Autodesk Fusion 360 part; units mm, degrees
(part 7 of 9)
  spline S163 degree 3 poles (2.1351, 29.8276) (2.5485, 29.4473) (2.7552, 28.9129) (2.7552, 28.2236) knots 0 0 0 0 1 1 1 1
  spline S164 degree 3 poles (2.7552, 28.2236) (2.7552, 27.6314) (2.5712, 27.1156) (2.2023, 26.6753) knots 0 0 0 0 1 1 1 1
  spline S165 degree 3 poles (2.2023, 26.6753) (1.8333, 26.2361) (1.2669, 26.017) (0.5021, 26.017) knots 0 0 0 0 1 1 1 1
  line L345 (0.5021, 26.017) -> (-1.8853, 26.017)
  line L346 (-1.8853, 26.017) -> (-1.8853, 22.8079)
  line L347 (-1.8853, 22.8079) -> (-2.9137, 22.8079)
  line L348 (-2.9137, 22.8079) -> (-2.9137, 30.3992)
  spline S166 degree 3 poles (1.7165, 28.2184) (1.7165, 28.7765) (1.5098, 29.1558) (1.0964, 29.3553) knots 0 0 0 0 1 1 1 1
  spline S167 degree 3 poles (1.0964, 29.3553) (0.869, 29.4617) (0.5569, 29.5155) (0.161, 29.5155) knots 0 0 0 0 1 1 1 1
  line L349 (0.161, 29.5155) -> (-1.8853, 29.5155)
  line L350 (-1.8853, 29.5155) -> (-1.8853, 26.8852)
  line L351 (-1.8853, 26.8852) -> (0.161, 26.8852)
  spline S168 degree 3 poles (0.161, 26.8852) (0.623, 26.8852) (0.9972, 26.9833) (1.2855, 27.1797) knots 0 0 0 0 1 1 1 1
  spline S169 degree 3 poles (1.2855, 27.1797) (1.5728, 27.3761) (1.7165, 27.7223) (1.7165, 28.2184) knots 0 0 0 0 1 1 1 1
  line L352 (13.755, 30.3992) -> (17.1709, 30.3992)
  spline S170 degree 3 poles (17.1709, 30.3992) (17.8458, 30.3992) (18.3904, 30.209) (18.8038, 29.8276) knots 0 0 0 0 1 1 1 1
  spline S171 degree 3 poles (18.8038, 29.8276) (19.2172, 29.4473) (19.424, 28.9129) (19.424, 28.2236) knots 0 0 0 0 1 1 1 1
  spline S172 degree 3 poles (19.424, 28.2236) (19.424, 27.6314) (19.24, 27.1156) (18.871, 26.6753) knots 0 0 0 0 1 1 1 1
  spline S173 degree 3 poles (18.871, 26.6753) (18.502, 26.2361) (17.9357, 26.017) (17.1709, 26.017) knots 0 0 0 0 1 1 1 1
  line L353 (17.1709, 26.017) -> (14.7834, 26.017)
  line L354 (14.7834, 26.017) -> (14.7834, 22.8079)
  line L355 (14.7834, 22.8079) -> (13.755, 22.8079)
  line L356 (13.755, 22.8079) -> (13.755, 30.3992)
  spline S174 degree 3 poles (18.3853, 28.2184) (18.3853, 28.7765) (18.1785, 29.1558) (17.7651, 29.3553) knots 0 0 0 0 1 1 1 1
  spline S175 degree 3 poles (17.7651, 29.3553) (17.5378, 29.4617) (17.2256, 29.5155) (16.8298, 29.5155) knots 0 0 0 0 1 1 1 1
  line L357 (16.8298, 29.5155) -> (14.7834, 29.5155)
  line L358 (14.7834, 29.5155) -> (14.7834, 26.8852)
  line L359 (14.7834, 26.8852) -> (16.8298, 26.8852)
  spline S176 degree 3 poles (16.8298, 26.8852) (17.2918, 26.8852) (17.6659, 26.9833) (17.9543, 27.1797) knots 0 0 0 0 1 1 1 1
  spline S177 degree 3 poles (17.9543, 27.1797) (18.2416, 27.3761) (18.3853, 27.7223) (18.3853, 28.2184) knots 0 0 0 0 1 1 1 1
  line L360 (29.7365, 30.3992) -> (30.9354, 30.3992)
  line L361 (30.9354, 30.3992) -> (33.1161, 26.7508)
  line L362 (33.1161, 26.7508) -> (35.2969, 30.3992)
  line L363 (35.2969, 30.3992) -> (36.5009, 30.3992)
  line L364 (36.5009, 30.3992) -> (33.6329, 25.8671)
  line L365 (33.6329, 25.8671) -> (33.6329, 22.8079)
  line L366 (33.6329, 22.8079) -> (32.6045, 22.8079)
  line L367 (32.6045, 22.8079) -> (32.6045, 25.8671)
  line L368 (32.6045, 25.8671) -> (29.7365, 30.3992)
  line L369 (47.5938, 30.3992) -> (49.7746, 23.9344)
  line L370 (49.7746, 23.9344) -> (51.9295, 30.3992)
  line L371 (51.9295, 30.3992) -> (53.0818, 30.3992)
  line L372 (53.0818, 30.3992) -> (50.312, 22.8079)
  line L373 (50.312, 22.8079) -> (49.2216, 22.8079)
  line L374 (49.2216, 22.8079) -> (46.4569, 30.3992)
  line L375 (46.4569, 30.3992) -> (47.5938, 30.3992)
  spline S178 degree 3 poles (66.3534, 30.6059) (67.6939, 30.6059) (68.6861, 30.1749) (69.3299, 29.3139) knots 0 0 0 0 1 1 1 1
  spline S179 degree 3 poles (69.3299, 29.3139) (69.8333, 28.6422) (70.0844, 27.7823) (70.0844, 26.7353) knots 0 0 0 0 1 1 1 1
  spline S180 degree 3 poles (70.0844, 26.7353) (70.0844, 25.6015) (69.7971, 24.66) (69.2214, 23.9086) knots 0 0 0 0 1 1 1 1
  spline S181 degree 3 poles (69.2214, 23.9086) (68.5465, 23.027) (67.5833, 22.5857) (66.3327, 22.5857) knots 0 0 0 0 1 1 1 1
  spline S182 degree 3 poles (66.3327, 22.5857) (65.1648, 22.5857) (64.2471, 22.9712) (63.5784, 23.7432) knots 0 0 0 0 1 1 1 1
  spline S183 degree 3 poles (63.5784, 23.7432) (62.982, 24.4874) (62.6844, 25.4279) (62.6844, 26.5648) knots 0 0 0 0 1 1 1 1
  spline S184 degree 3 poles (62.6844, 26.5648) (62.6844, 27.5911) (62.9396, 28.4696) (63.4492, 29.2003) knots 0 0 0 0 1 1 1 1
  spline S185 degree 3 poles (63.4492, 29.2003) (64.1034, 30.1377) (65.0718, 30.6059) (66.3534, 30.6059) knots 0 0 0 0 1 1 1 1
  spline S186 degree 3 poles (66.4567, 23.5055) (67.3631, 23.5055) (68.0184, 23.83) (68.4225, 24.4801) knots 0 0 0 0 1 1 1 1
  spline S187 degree 3 poles (68.4225, 24.4801) (68.8277, 25.1292) (69.0302, 25.8754) (69.0302, 26.7198) knots 0 0 0 0 1 1 1 1
  spline S188 degree 3 poles (69.0302, 26.7198) (69.0302, 27.6117) (68.7966, 28.33) (68.3295, 28.8747) knots 0 0 0 0 1 1 1 1
  spline S189 degree 3 poles (68.3295, 28.8747) (67.8634, 29.4194) (67.2247, 29.6912) (66.4154, 29.6912) knots 0 0 0 0 1 1 1 1
  spline S190 degree 3 poles (66.4154, 29.6912) (65.6299, 29.6912) (64.9891, 29.4214) (64.493, 28.883) knots 0 0 0 0 1 1 1 1
  spline S191 degree 3 poles (64.493, 28.883) (63.9969, 28.3435) (63.7489, 27.5487) (63.7489, 26.4976) knots 0 0 0 0 1 1 1 1
  spline S192 degree 3 poles (63.7489, 26.4976) (63.7489, 25.6573) (63.9618, 24.9483) (64.3876, 24.3706) knots 0 0 0 0 1 1 1 1
  spline S193 degree 3 poles (64.3876, 24.3706) (64.8124, 23.7939) (65.5028, 23.5055) (66.4567, 23.5055) knots 0 0 0 0 1 1 1 1
  spline S194 degree 3 poles (83.5689, 26.9213) (84.0515, 26.9213) (84.4329, 27.0174) (84.713, 27.2107) knots 0 0 0 0 1 1 1 1
  spline S195 degree 3 poles (84.713, 27.2107) (84.9941, 27.404) (85.1347, 27.7513) (85.1347, 28.2546) knots 0 0 0 0 1 1 1 1
  spline S196 degree 3 poles (85.1347, 28.2546) (85.1347, 28.7951) (84.9383, 29.1641) (84.5456, 29.3605) knots 0 0 0 0 1 1 1 1
  spline S197 degree 3 poles (84.5456, 29.3605) (84.3358, 29.4638) (84.0546, 29.5155) (83.7032, 29.5155) knots 0 0 0 0 1 1 1 1
  line L376 (83.7032, 29.5155) -> (81.1918, 29.5155)
  line L377 (81.1918, 29.5155) -> (81.1918, 26.9213)
  line L378 (81.1918, 26.9213) -> (83.5689, 26.9213)
  line L379 (80.1634, 30.3992) -> (83.6774, 30.3992)
  spline S198 degree 3 poles (83.6774, 30.3992) (84.2562, 30.3992) (84.7337, 30.3144) (85.1088, 30.1459) knots 0 0 0 0 1 1 1 1
  spline S199 degree 3 poles (85.1088, 30.1459) (85.822, 29.8224) (86.1785, 29.224) (86.1785, 28.3528) knots 0 0 0 0 1 1 1 1
  spline S200 degree 3 poles (86.1785, 28.3528) (86.1785, 27.898) (86.0845, 27.5259) (85.8974, 27.2366) knots 0 0 0 0 1 1 1 1
  spline S201 degree 3 poles (85.8974, 27.2366) (85.7093, 26.9472) (85.4468, 26.7146) (85.1088, 26.5389) knots 0 0 0 0 1 1 1 1
  spline S202 degree 3 poles (85.1088, 26.5389) (85.4055, 26.418) (85.6287, 26.2599) (85.7775, 26.0635) knots 0 0 0 0 1 1 1 1
  spline S203 degree 3 poles (85.7775, 26.0635) (85.9274, 25.8671) (86.0111, 25.5488) (86.0287, 25.1075) knots 0 0 0 0 1 1 1 1
  line L380 (86.0287, 25.1075) -> (86.0648, 24.0895)
  spline S204 degree 3 poles (86.0648, 24.0895) (86.0752, 23.8001) (86.099, 23.5851) (86.1372, 23.4435) knots 0 0 0 0 1 1 1 1
  spline S205 degree 3 poles (86.1372, 23.4435) (86.1992, 23.2027) (86.3098, 23.0477) (86.4679, 22.9784) knots 0 0 0 0 1 1 1 1
  line L381 (86.4679, 22.9784) -> (86.4679, 22.8079)
  line L382 (86.4679, 22.8079) -> (85.207, 22.8079)
  spline S206 degree 3 poles (85.207, 22.8079) (85.1729, 22.873) (85.145, 22.9577) (85.1243, 23.0611) knots 0 0 0 0 1 1 1 1
  spline S207 degree 3 poles (85.1243, 23.0611) (85.1037, 23.1645) (85.0861, 23.3639) (85.0727, 23.6605) knots 0 0 0 0 1 1 1 1
  line L383 (85.0727, 23.6605) -> (85.0106, 24.9266)
  spline S208 degree 3 poles (85.0106, 24.9266) (84.9869, 25.4227) (84.8019, 25.7555) (84.4577, 25.924) knots 0 0 0 0 1 1 1 1
  spline S209 degree 3 poles (84.4577, 25.924) (84.2613, 26.017) (83.9533, 26.0635) (83.5327, 26.0635) knots 0 0 0 0 1 1 1 1
  line L384 (83.5327, 26.0635) -> (81.1918, 26.0635)
  line L385 (81.1918, 26.0635) -> (81.1918, 22.8079)
  line L386 (81.1918, 22.8079) -> (80.1634, 22.8079)
  line L387 (80.1634, 22.8079) -> (80.1634, 30.3992)
  line L388 (-86.6223, 11.899) -> (-85.5836, 11.899)
  line L389 (-85.5836, 11.899) -> (-85.5836, 8.7622)
  line L390 (-85.5836, 8.7622) -> (-81.6355, 8.7622)
  line L391 (-81.6355, 8.7622) -> (-81.6355, 11.899)
  line L392 (-81.6355, 11.899) -> (-80.5968, 11.899)
  line L393 (-80.5968, 11.899) -> (-80.5968, 4.3077)
  line L394 (-80.5968, 4.3077) -> (-81.6355, 4.3077)
  line L395 (-81.6355, 4.3077) -> (-81.6355, 7.8579)
  line L396 (-81.6355, 7.8579) -> (-85.5836, 7.8579)
  line L397 (-85.5836, 7.8579) -> (-85.5836, 4.3077)
  line L398 (-85.5836, 4.3077) -> (-86.6223, 4.3077)
  line L399 (-86.6223, 4.3077) -> (-86.6223, 11.899)
  line L400 (-65.7905, 7.4186) -> (-66.9429, 10.7724)
  line L401 (-66.9429, 10.7724) -> (-68.1676, 7.4186)
  line L402 (-68.1676, 7.4186) -> (-65.7905, 7.4186)
  line L403 (-67.4803, 11.899) -> (-66.3176, 11.899)
  line L404 (-66.3176, 11.899) -> (-63.5632, 4.3077)
  line L405 (-63.5632, 4.3077) -> (-64.6898, 4.3077)
  line L406 (-64.6898, 4.3077) -> (-65.4598, 6.5815)
  line L407 (-65.4598, 6.5815) -> (-68.4622, 6.5815)
  line L408 (-68.4622, 6.5815) -> (-69.2838, 4.3077)
  line L409 (-69.2838, 4.3077) -> (-70.338, 4.3077)
  line L410 (-70.338, 4.3077) -> (-67.4803, 11.899)
  line L411 (-52.4321, 11.899) -> (-51.4038, 11.899)
  line L412 (-51.4038, 11.899) -> (-51.4038, 5.2121)
  line L413 (-51.4038, 5.2121) -> (-47.559, 5.2121)
  line L414 (-47.559, 5.2121) -> (-47.559, 4.3077)
  line L415 (-47.559, 4.3077) -> (-52.4321, 4.3077)
  line L416 (-52.4321, 4.3077) -> (-52.4321, 11.899)
  spline S210 degree 3 poles (-33.4969, 8.6899) (-33.0628, 8.6899) (-32.7248, 8.7498) (-32.484, 8.8708) knots 0 0 0 0 1 1 1 1
  spline S211 degree 3 poles (-32.484, 8.8708) (-32.1047, 9.0599) (-31.9156, 9.401) (-31.9156, 9.8939) knots 0 0 0 0 1 1 1 1
  spline S212 degree 3 poles (-31.9156, 9.8939) (-31.9156, 10.39) (-32.1171, 10.7239) (-32.5202, 10.8965) knots 0 0 0 0 1 1 1 1
  spline S213 degree 3 poles (-32.5202, 10.8965) (-32.7475, 10.9926) (-33.0855, 11.0412) (-33.533, 11.0412) knots 0 0 0 0 1 1 1 1
  line L417 (-33.533, 11.0412) -> (-35.3675, 11.0412)
  line L418 (-35.3675, 11.0412) -> (-35.3675, 8.6899)
  line L419 (-35.3675, 8.6899) -> (-33.4969, 8.6899)
  spline S214 degree 3 poles (-33.1506, 5.1862) (-32.5202, 5.1862) (-32.0706, 5.3692) (-31.8019, 5.734) knots 0 0 0 0 1 1 1 1
  spline S215 degree 3 poles (-31.8019, 5.734) (-31.6334, 5.9645) (-31.5486, 6.2435) (-31.5486, 6.5712) knots 0 0 0 0 1 1 1 1
  spline S216 degree 3 poles (-31.5486, 6.5712) (-31.5486, 7.122) (-31.7946, 7.4982) (-32.2876, 7.6977) knots 0 0 0 0 1 1 1 1
  spline S217 degree 3 poles (-32.2876, 7.6977) (-32.5491, 7.8042) (-32.8953, 7.8579) (-33.3263, 7.8579) knots 0 0 0 0 1 1 1 1
  line L420 (-33.3263, 7.8579) -> (-35.3675, 7.8579)
  line L421 (-35.3675, 7.8579) -> (-35.3675, 5.1862)
  line L422 (-35.3675, 5.1862) -> (-33.1506, 5.1862)
  line L423 (-36.3752, 11.899) -> (-33.1144, 11.899)
  spline S218 degree 3 poles (-33.1144, 11.899) (-32.2256, 11.899) (-31.5931, 11.6334) (-31.2179, 11.1032) knots 0 0 0 0 1 1 1 1
  spline S219 degree 3 poles (-31.2179, 11.1032) (-30.9978, 10.79) (-30.8872, 10.4283) (-30.8872, 10.018) knots 0 0 0 0 1 1 1 1
  spline S220 degree 3 poles (-30.8872, 10.018) (-30.8872, 9.5394) (-31.0236, 9.1467) (-31.2954, 8.8397) knots 0 0 0 0 1 1 1 1
  spline S221 degree 3 poles (-31.2954, 8.8397) (-31.437, 8.6775) (-31.6396, 8.5297) (-31.9052, 8.3953) knots 0 0 0 0 1 1 1 1
  spline S222 degree 3 poles (-31.9052, 8.3953) (-31.5156, 8.2475) (-31.2252, 8.0801) (-31.0319, 7.8941) knots 0 0 0 0 1 1 1 1
  spline S223 degree 3 poles (-31.0319, 7.8941) (-30.6908, 7.5633) (-30.5203, 7.1065) (-30.5203, 6.5246) knots 0 0 0 0 1 1 1 1
  spline S224 degree 3 poles (-30.5203, 6.5246) (-30.5203, 6.0358) (-30.6733, 5.5924) (-30.9802, 5.1966) knots 0 0 0 0 1 1 1 1
  spline S225 degree 3 poles (-30.9802, 5.1966) (-31.4381, 4.6043) (-32.1667, 4.3077) (-33.1661, 4.3077) knots 0 0 0 0 1 1 1 1
  line L424 (-33.1661, 4.3077) -> (-36.3752, 4.3077)
  line L425 (-36.3752, 4.3077) -> (-36.3752, 11.899)
  line L426 (-17.3883, 11.899) -> (-16.3496, 11.899)
  line L427 (-16.3496, 11.899) -> (-16.3496, 4.3077)
  line L428 (-16.3496, 4.3077) -> (-17.3883, 4.3077)
  line L429 (-17.3883, 4.3077) -> (-17.3883, 11.899)
  spline S226 degree 3 poles (0.2251, 8.4212) (0.7078, 8.4212) (1.0892, 8.5173) (1.3692, 8.7106) knots 0 0 0 0 1 1 1 1
  spline S227 degree 3 poles (1.3692, 8.7106) (1.6504, 8.9038) (1.7909, 9.2511) (1.7909, 9.7544) knots 0 0 0 0 1 1 1 1
  spline S228 degree 3 poles (1.7909, 9.7544) (1.7909, 10.295) (1.5945, 10.6639) (1.2018, 10.8603) knots 0 0 0 0 1 1 1 1
  spline S229 degree 3 poles (1.2018, 10.8603) (0.992, 10.9636) (0.7109, 11.0153) (0.3595, 11.0153) knots 0 0 0 0 1 1 1 1
  line L430 (0.3595, 11.0153) -> (-2.152, 11.0153)
  line L431 (-2.152, 11.0153) -> (-2.152, 8.4212)
  line L432 (-2.152, 8.4212) -> (0.2251, 8.4212)
  line L433 (-3.1804, 11.899) -> (0.3336, 11.899)
  spline S230 degree 3 poles (0.3336, 11.899) (0.9124, 11.899) (1.3899, 11.8142) (1.7651, 11.6458) knots 0 0 0 0 1 1 1 1
  spline S231 degree 3 poles (1.7651, 11.6458) (2.4782, 11.3223) (2.8348, 10.7239) (2.8348, 9.8526) knots 0 0 0 0 1 1 1 1
  spline S232 degree 3 poles (2.8348, 9.8526) (2.8348, 9.3979) (2.7407, 9.0258) (2.5537, 8.7364) knots 0 0 0 0 1 1 1 1
  spline S233 degree 3 poles (2.5537, 8.7364) (2.3656, 8.447) (2.103, 8.2145) (1.7651, 8.0388) knots 0 0 0 0 1 1 1 1
  spline S234 degree 3 poles (1.7651, 8.0388) (2.0617, 7.9178) (2.2849, 7.7597) (2.4338, 7.5633) knots 0 0 0 0 1 1 1 1
  spline S235 degree 3 poles (2.4338, 7.5633) (2.5836, 7.367) (2.6674, 7.0486) (2.6849, 6.6073) knots 0 0 0 0 1 1 1 1
  line L434 (2.6849, 6.6073) -> (2.7211, 5.5893)
  spline S236 degree 3 poles (2.7211, 5.5893) (2.7314, 5.2999) (2.7552, 5.0849) (2.7934, 4.9433) knots 0 0 0 0 1 1 1 1
  spline S237 degree 3 poles (2.7934, 4.9433) (2.8555, 4.7025) (2.966, 4.5475) (3.1242, 4.4783) knots 0 0 0 0 1 1 1 1
  line L435 (3.1242, 4.4783) -> (3.1242, 4.3077)
  line L436 (3.1242, 4.3077) -> (1.8633, 4.3077)
  spline S238 degree 3 poles (1.8633, 4.3077) (1.8292, 4.3728) (1.8013, 4.4576) (1.7806, 4.5609) knots 0 0 0 0 1 1 1 1
  spline S239 degree 3 poles (1.7806, 4.5609) (1.7599, 4.6643) (1.7423, 4.8638) (1.7289, 5.1604) knots 0 0 0 0 1 1 1 1
  line L437 (1.7289, 5.1604) -> (1.6669, 6.4265)
  spline S240 degree 3 poles (1.6669, 6.4265) (1.6431, 6.9226) (1.4581, 7.2553) (1.114, 7.4238) knots 0 0 0 0 1 1 1 1
  spline S241 degree 3 poles (1.114, 7.4238) (0.9176, 7.5168) (0.6096, 7.5633) (0.1889, 7.5633) knots 0 0 0 0 1 1 1 1
  line L438 (0.1889, 7.5633) -> (-2.152, 7.5633)
  line L439 (-2.152, 7.5633) -> (-2.152, 4.3077)
  line L440 (-2.152, 4.3077) -> (-3.1804, 4.3077)
  line L441 (-3.1804, 4.3077) -> (-3.1804, 11.899)
  line L442 (19.4777, 11.899) -> (19.4777, 10.9947)
  line L443 (19.4777, 10.9947) -> (16.9197, 10.9947)
  line L444 (16.9197, 10.9947) -> (16.9197, 4.3077)
  line L445 (16.9197, 4.3077) -> (15.8758, 4.3077)
  line L446 (15.8758, 4.3077) -> (15.8758, 10.9947)
  line L447 (15.8758, 10.9947) -> (13.3179, 10.9947)
  line L448 (13.3179, 10.9947) -> (13.3179, 11.899)
  line L449 (13.3179, 11.899) -> (19.4777, 11.899)
  line L450 (30.059, 11.899) -> (31.0977, 11.899)
  line L451 (31.0977, 11.899) -> (31.0977, 8.7622)
  line L452 (31.0977, 8.7622) -> (35.0457, 8.7622)
  line L453 (35.0457, 8.7622) -> (35.0457, 11.899)
  line L454 (35.0457, 11.899) -> (36.0844, 11.899)
  line L455 (36.0844, 11.899) -> (36.0844, 4.3077)
  line L456 (36.0844, 4.3077) -> (35.0457, 4.3077)
  line L457 (35.0457, 4.3077) -> (35.0457, 7.8579)
  line L458 (35.0457, 7.8579) -> (31.0977, 7.8579)
  line L459 (31.0977, 7.8579) -> (31.0977, 4.3077)
  line L460 (31.0977, 4.3077) -> (30.059, 4.3077)
  line L461 (30.059, 4.3077) -> (30.059, 11.899)
  spline S242 degree 3 poles (49.6164, 5.1862) (49.9647, 5.1862) (50.25, 5.2224) (50.4743, 5.2947) knots 0 0 0 0 1 1 1 1
  spline S243 degree 3 poles (50.4743, 5.2947) (50.8742, 5.4291) (51.2008, 5.6875) (51.4561, 6.0699) knots 0 0 0 0 1 1 1 1
  spline S244 degree 3 poles (51.4561, 6.0699) (51.6597, 6.3768) (51.8054, 6.7696) (51.8954, 7.2481) knots 0 0 0 0 1 1 1 1
  spline S245 degree 3 poles (51.8954, 7.2481) (51.947, 7.5344) (51.9729, 7.799) (51.9729, 8.0439) knots 0 0 0 0 1 1 1 1
  spline S246 degree 3 poles (51.9729, 8.0439) (51.9729, 8.9844) (51.7858, 9.7151) (51.4127, 10.235) knots 0 0 0 0 1 1 1 1
  spline S247 degree 3 poles (51.4127, 10.235) (51.0386, 10.7549) (50.436, 11.0153) (49.6061, 11.0153) knots 0 0 0 0 1 1 1 1
  line L462 (49.6061, 11.0153) -> (47.7819, 11.0153)
  line L463 (47.7819, 11.0153) -> (47.7819, 5.1862)
  line L464 (47.7819, 5.1862) -> (49.6164, 5.1862)
  line L465 (46.7484, 11.899) -> (49.8231, 11.899)
  spline S248 degree 3 poles (49.8231, 11.899) (50.867, 11.899) (51.6762, 11.529) (52.2519, 10.7879) knots 0 0 0 0 1 1 1 1
  spline S249 degree 3 poles (52.2519, 10.7879) (52.7656, 10.1193) (53.0219, 9.2635) (53.0219, 8.2196) knots 0 0 0 0 1 1 1 1
  spline S250 degree 3 poles (53.0219, 8.2196) (53.0219, 7.4135) (52.87, 6.6848) (52.5671, 6.0337) knots 0 0 0 0 1 1 1 1
  spline S251 degree 3 poles (52.5671, 6.0337) (52.0328, 4.8834) (51.115, 4.3077) (49.8128, 4.3077) knots 0 0 0 0 1 1 1 1
  line L466 (49.8128, 4.3077) -> (46.7484, 4.3077)
  line L467 (46.7484, 4.3077) -> (46.7484, 11.899)
  line L468 (67.5595, 7.4186) -> (66.4071, 10.7724)
  line L469 (66.4071, 10.7724) -> (65.1824, 7.4186)
  line L470 (65.1824, 7.4186) -> (67.5595, 7.4186)
  line L471 (65.8697, 11.899) -> (67.0324, 11.899)
  line L472 (67.0324, 11.899) -> (69.7868, 4.3077)
  line L473 (69.7868, 4.3077) -> (68.6602, 4.3077)
  line L474 (68.6602, 4.3077) -> (67.8902, 6.5815)
  line L475 (67.8902, 6.5815) -> (64.8878, 6.5815)
  line L476 (64.8878, 6.5815) -> (64.0662, 4.3077)
  line L477 (64.0662, 4.3077) -> (63.012, 4.3077)
  line L478 (63.012, 4.3077) -> (65.8697, 11.899)
  line L479 (79.7427, 11.899) -> (80.9416, 11.899)
  line L480 (80.9416, 11.899) -> (83.1224, 8.2506)
  line L481 (83.1224, 8.2506) -> (85.3031, 11.899)
  line L482 (85.3031, 11.899) -> (86.5072, 11.899)
  line L483 (86.5072, 11.899) -> (83.6392, 7.367)
  line L484 (83.6392, 7.367) -> (83.6392, 4.3077)
  line L485 (83.6392, 4.3077) -> (82.6108, 4.3077)
  line L486 (82.6108, 4.3077) -> (82.6108, 7.367)
  line L487 (82.6108, 7.367) -> (79.7427, 11.899)
  spline S252 degree 3 poles (-83.7336, -13.3139) (-83.3853, -13.3139) (-83.1, -13.2778) (-82.8757, -13.2054) knots 0 0 0 0 1 1 1 1
  spline S253 degree 3 poles (-82.8757, -13.2054) (-82.4758, -13.0711) (-82.1492, -12.8127) (-81.8939, -12.4303) knots 0 0 0 0 1 1 1 1
  spline S254 degree 3 poles (-81.8939, -12.4303) (-81.6903, -12.1233) (-81.5446, -11.7306) (-81.4546, -11.2521) knots 0 0 0 0 1 1 1 1
  spline S255 degree 3 poles (-81.4546, -11.2521) (-81.403, -10.9658) (-81.3771, -10.7012) (-81.3771, -10.4562) knots 0 0 0 0 1 1 1 1
  spline S256 degree 3 poles (-81.3771, -10.4562) (-81.3771, -9.5157) (-81.5642, -8.785) (-81.9373, -8.2652) knots 0 0 0 0 1 1 1 1
  spline S257 degree 3 poles (-81.9373, -8.2652) (-82.3114, -7.7453) (-82.914, -7.4848) (-83.7439, -7.4848) knots 0 0 0 0 1 1 1 1
  line L488 (-83.7439, -7.4848) -> (-85.5681, -7.4848)
  line L489 (-85.5681, -7.4848) -> (-85.5681, -13.3139)
  line L490 (-85.5681, -13.3139) -> (-83.7336, -13.3139)
  line L491 (-86.6016, -6.6012) -> (-83.5269, -6.6012)
  spline S258 degree 3 poles (-83.5269, -6.6012) (-82.483, -6.6012) (-81.6738, -6.9712) (-81.0981, -7.7122) knots 0 0 0 0 1 1 1 1
  spline S259 degree 3 poles (-81.0981, -7.7122) (-80.5844, -8.3809) (-80.3281, -9.2367) (-80.3281, -10.2805) knots 0 0 0 0 1 1 1 1
  spline S260 degree 3 poles (-80.3281, -10.2805) (-80.3281, -11.0867) (-80.48, -11.8153) (-80.7829, -12.4664) knots 0 0 0 0 1 1 1 1
  spline S261 degree 3 poles (-80.7829, -12.4664) (-81.3172, -13.6168) (-82.235, -14.1924) (-83.5372, -14.1924) knots 0 0 0 0 1 1 1 1
  line L492 (-83.5372, -14.1924) -> (-86.6016, -14.1924)
  line L493 (-86.6016, -14.1924) -> (-86.6016, -6.6012)
  spline S262 degree 3 poles (-66.4499, -10.079) (-65.9672, -10.079) (-65.5858, -9.9829) (-65.3058, -9.7896) knots 0 0 0 0 1 1 1 1
  spline S263 degree 3 poles (-65.3058, -9.7896) (-65.0246, -9.5963) (-64.8841, -9.2491) (-64.8841, -8.7457) knots 0 0 0 0 1 1 1 1
  spline S264 degree 3 poles (-64.8841, -8.7457) (-64.8841, -8.2052) (-65.0805, -7.8362) (-65.4732, -7.6399) knots 0 0 0 0 1 1 1 1
  spline S265 degree 3 poles (-65.4732, -7.6399) (-65.683, -7.5365) (-65.9641, -7.4848) (-66.3155, -7.4848) knots 0 0 0 0 1 1 1 1
  line L494 (-66.3155, -7.4848) -> (-68.827, -7.4848)
  line L495 (-68.827, -7.4848) -> (-68.827, -10.079)
  line L496 (-68.827, -10.079) -> (-66.4499, -10.079)
  line L497 (-69.8554, -6.6012) -> (-66.3414, -6.6012)
  spline S266 degree 3 poles (-66.3414, -6.6012) (-65.7626, -6.6012) (-65.2851, -6.6859) (-64.9099, -6.8544) knots 0 0 0 0 1 1 1 1
  spline S267 degree 3 poles (-64.9099, -6.8544) (-64.1968, -7.1779) (-63.8402, -7.7763) (-63.8402, -8.6476) knots 0 0 0 0 1 1 1 1
  spline S268 degree 3 poles (-63.8402, -8.6476) (-63.8402, -9.1023) (-63.9343, -9.4744) (-64.1213, -9.7638) knots 0 0 0 0 1 1 1 1
  spline S269 degree 3 poles (-64.1213, -9.7638) (-64.3094, -10.0532) (-64.572, -10.2857) (-64.9099, -10.4614) knots 0 0 0 0 1 1 1 1
  spline S270 degree 3 poles (-64.9099, -10.4614) (-64.6133, -10.5823) (-64.3901, -10.7405) (-64.2412, -10.9368) knots 0 0 0 0 1 1 1 1
  spline S271 degree 3 poles (-64.2412, -10.9368) (-64.0914, -11.1332) (-64.0076, -11.4515) (-63.9901, -11.8928) knots 0 0 0 0 1 1 1 1
  line L498 (-63.9901, -11.8928) -> (-63.9539, -12.9109)
  spline S272 degree 3 poles (-63.9539, -12.9109) (-63.9436, -13.2003) (-63.9198, -13.4152) (-63.8816, -13.5568) knots 0 0 0 0 1 1 1 1
  spline S273 degree 3 poles (-63.8816, -13.5568) (-63.8195, -13.7976) (-63.709, -13.9527) (-63.5508, -14.0219) knots 0 0 0 0 1 1 1 1
  line L499 (-63.5508, -14.0219) -> (-63.5508, -14.1924)
  line L500 (-63.5508, -14.1924) -> (-64.8117, -14.1924)
  spline S274 degree 3 poles (-64.8117, -14.1924) (-64.8458, -14.1273) (-64.8737, -14.0426) (-64.8944, -13.9392) knots 0 0 0 0 1 1 1 1
  spline S275 degree 3 poles (-64.8944, -13.9392) (-64.9151, -13.8359) (-64.9327, -13.6364) (-64.9461, -13.3398) knots 0 0 0 0 1 1 1 1
  line L501 (-64.9461, -13.3398) -> (-65.0081, -12.0737)
  spline S276 degree 3 poles (-65.0081, -12.0737) (-65.0319, -11.5776) (-65.2169, -11.2448) (-65.561, -11.0764) knots 0 0 0 0 1 1 1 1
  spline S277 degree 3 poles (-65.561, -11.0764) (-65.7574, -10.9833) (-66.0654, -10.9368) (-66.4861, -10.9368) knots 0 0 0 0 1 1 1 1
  line L502 (-66.4861, -10.9368) -> (-68.827, -10.9368)
  line L503 (-68.827, -10.9368) -> (-68.827, -14.1924)
  line L504 (-68.827, -14.1924) -> (-69.8554, -14.1924)
  line L505 (-69.8554, -14.1924) -> (-69.8554, -6.6012)
  line L506 (-53.2848, -13.3398) -> (-48.6287, -7.5055)
  line L507 (-48.6287, -7.5055) -> (-52.9437, -7.5055)
  line L508 (-52.9437, -7.5055) -> (-52.9437, -6.6012)
  line L509 (-52.9437, -6.6012) -> (-47.3058, -6.6012)
  line L510 (-47.3058, -6.6012) -> (-47.3058, -7.4848)
  line L511 (-47.3058, -7.4848) -> (-51.9877, -13.2881)
  line L512 (-51.9877, -13.2881) -> (-47.3058, -13.2881)
  line L513 (-47.3058, -13.2881) -> (-47.3058, -14.1924)
  line L514 (-47.3058, -14.1924) -> (-53.2848, -14.1924)
  line L515 (-53.2848, -14.1924) -> (-53.2848, -13.3398)
  line L516 (-37.3126, -6.6012) -> (-35.8812, -12.7765)
  line L517 (-35.8812, -12.7765) -> (-34.1655, -6.6012)
  line L518 (-34.1655, -6.6012) -> (-33.0493, -6.6012)
  line L519 (-33.0493, -6.6012) -> (-31.3337, -12.7765)
  line L520 (-31.3337, -12.7765) -> (-29.9022, -6.6012)
  line L521 (-29.9022, -6.6012) -> (-28.7757, -6.6012)
  line L522 (-28.7757, -6.6012) -> (-30.7704, -14.1924)
  line L523 (-30.7704, -14.1924) -> (-31.8504, -14.1924)
  line L524 (-31.8504, -14.1924) -> (-33.6023, -7.8983)
  line L525 (-33.6023, -7.8983) -> (-35.3644, -14.1924)
  line L526 (-35.3644, -14.1924) -> (-36.4445, -14.1924)
  line L527 (-36.4445, -14.1924) -> (-38.4288, -6.6012)
  line L528 (-38.4288, -6.6012) -> (-37.3126, -6.6012)
  spline S278 degree 3 poles (-16.9904, -6.3945) (-15.6499, -6.3945) (-14.6577, -6.8254) (-14.0138, -7.6864) knots 0 0 0 0 1 1 1 1
  spline S279 degree 3 poles (-14.0138, -7.6864) (-13.5105, -8.3582) (-13.2593, -9.2181) (-13.2593, -10.265) knots 0 0 0 0 1 1 1 1
  spline S280 degree 3 poles (-13.2593, -10.265) (-13.2593, -11.3988) (-13.5466, -12.3404) (-14.1223, -13.0917) knots 0 0 0 0 1 1 1 1
  spline S281 degree 3 poles (-14.1223, -13.0917) (-14.7972, -13.9733) (-15.7605, -14.4146) (-17.011, -14.4146) knots 0 0 0 0 1 1 1 1
  spline S282 degree 3 poles (-17.011, -14.4146) (-18.1789, -14.4146) (-19.0967, -14.0291) (-19.7654, -13.2571) knots 0 0 0 0 1 1 1 1
  spline S283 degree 3 poles (-19.7654, -13.2571) (-20.3617, -12.513) (-20.6594, -11.5724) (-20.6594, -10.4356) knots 0 0 0 0 1 1 1 1
  spline S284 degree 3 poles (-20.6594, -10.4356) (-20.6594, -9.4093) (-20.4041, -8.5308) (-19.8946, -7.8001) knots 0 0 0 0 1 1 1 1
  spline S285 degree 3 poles (-19.8946, -7.8001) (-19.2404, -6.8627) (-18.2719, -6.3945) (-16.9904, -6.3945) knots 0 0 0 0 1 1 1 1
  spline S286 degree 3 poles (-16.887, -13.4948) (-15.9806, -13.4948) (-15.3253, -13.1703) (-14.9212, -12.5202) knots 0 0 0 0 1 1 1 1
  spline S287 degree 3 poles (-14.9212, -12.5202) (-14.5161, -11.8711) (-14.3135, -11.1249) (-14.3135, -10.2805) knots 0 0 0 0 1 1 1 1
  spline S288 degree 3 poles (-14.3135, -10.2805) (-14.3135, -9.3886) (-14.5471, -8.6703) (-15.0143, -8.1256) knots 0 0 0 0 1 1 1 1
  spline S289 degree 3 poles (-15.0143, -8.1256) (-15.4804, -7.581) (-16.1191, -7.3091) (-16.9284, -7.3091) knots 0 0 0 0 1 1 1 1
  spline S290 degree 3 poles (-16.9284, -7.3091) (-17.7138, -7.3091) (-18.3546, -7.5789) (-18.8507, -8.1174) knots 0 0 0 0 1 1 1 1
  spline S291 degree 3 poles (-18.8507, -8.1174) (-19.3468, -8.6569) (-19.5949, -9.4516) (-19.5949, -10.5027) knots 0 0 0 0 1 1 1 1
  spline S292 degree 3 poles (-19.5949, -10.5027) (-19.5949, -11.343) (-19.3819, -12.052) (-18.9561, -12.6297) knots 0 0 0 0 1 1 1 1
  spline S293 degree 3 poles (-18.9561, -12.6297) (-18.5314, -13.2065) (-17.841, -13.4948) (-16.887, -13.4948) knots 0 0 0 0 1 1 1 1
  line L529 (-16.4736, -4.5961) -> (-15.5073, -4.5961)
  line L530 (-15.5073, -4.5961) -> (-15.5073, -5.671)
  line L531 (-15.5073, -5.671) -> (-16.4736, -5.671)
  line L532 (-16.4736, -5.671) -> (-16.4736, -4.5961)
  line L533 (-18.1789, -4.5961) -> (-17.2126, -4.5961)
  line L534 (-17.2126, -4.5961) -> (-17.2126, -5.671)
  line L535 (-17.2126, -5.671) -> (-18.1789, -5.671)
  line L536 (-18.1789, -5.671) -> (-18.1789, -4.5961)
  line L537 (-2.4259, -6.6012) -> (-1.3975, -6.6012)
  line L538 (-1.3975, -6.6012) -> (-1.3975, -13.2881)
  line L539 (-1.3975, -13.2881) -> (2.4472, -13.2881)
  line L540 (2.4472, -13.2881) -> (2.4472, -14.1924)
  line L541 (2.4472, -14.1924) -> (-2.4259, -14.1924)
  line L542 (-2.4259, -14.1924) -> (-2.4259, -6.6012)
  line L543 (14.0517, -6.6012) -> (19.3175, -6.6012)
  line L544 (19.3175, -6.6012) -> (19.3175, -7.5313)
  line L545 (19.3175, -7.5313) -> (15.08, -7.5313)
  line L546 (15.08, -7.5313) -> (15.08, -9.8361)
  line L547 (15.08, -9.8361) -> (18.8059, -9.8361)
  line L548 (18.8059, -9.8361) -> (18.8059, -10.7405)
  line L549 (18.8059, -10.7405) -> (15.08, -10.7405)
  line L550 (15.08, -10.7405) -> (15.08, -14.1924)
  line L551 (15.08, -14.1924) -> (14.0517, -14.1924)
  line L552 (14.0517, -14.1924) -> (14.0517, -6.6012)
  line L553 (31.1493, -6.6012) -> (31.1493, -11.2934)
  spline S294 degree 3 poles (31.1493, -11.2934) (31.1493, -11.8443) (31.2527, -12.3031) (31.4594, -12.668) knots 0 0 0 0 1 1 1 1
  spline S295 degree 3 poles (31.4594, -12.668) (31.7663, -13.2189) (32.2831, -13.4948) (33.0097, -13.4948) knots 0 0 0 0 1 1 1 1
  spline S296 degree 3 poles (33.0097, -13.4948) (33.8809, -13.4948) (34.4742, -13.1972) (34.7874, -12.6008) knots 0 0 0 0 1 1 1 1
  spline S297 degree 3 poles (34.7874, -12.6008) (34.9558, -12.2773) (35.0406, -11.8412) (35.0406, -11.2934) knots 0 0 0 0 1 1 1 1
  line L554 (35.0406, -11.2934) -> (35.0406, -6.6012)
  line L555 (35.0406, -6.6012) -> (36.0844, -6.6012)
  line L556 (36.0844, -6.6012) -> (36.0844, -10.8645)
  spline S298 degree 3 poles (36.0844, -10.8645) (36.0844, -11.7978) (35.9583, -12.5161) (35.7072, -13.0194) knots 0 0 0 0 1 1 1 1
  spline S299 degree 3 poles (35.7072, -13.0194) (35.2452, -13.9361) (34.3739, -14.394) (33.0924, -14.394) knots 0 0 0 0 1 1 1 1
  spline S300 degree 3 poles (33.0924, -14.394) (31.8108, -14.394) (30.9406, -13.9361) (30.4827, -13.0194) knots 0 0 0 0 1 1 1 1
  spline S301 degree 3 poles (30.4827, -13.0194) (30.2316, -12.5161) (30.1055, -11.7978) (30.1055, -10.8645) knots 0 0 0 0 1 1 1 1
  line L557 (30.1055, -10.8645) -> (30.1055, -6.6012)
  line L558 (30.1055, -6.6012) -> (31.1493, -6.6012)
  line L559 (33.5833, -4.8028) -> (34.5496, -4.8028)
  line L560 (34.5496, -4.8028) -> (34.5496, -5.8777)
  line L561 (34.5496, -5.8777) -> (33.5833, -5.8777)
  line L562 (33.5833, -5.8777) -> (33.5833, -4.8028)
  line L563 (31.878, -4.8028) -> (32.8443, -4.8028)
  line L564 (32.8443, -4.8028) -> (32.8443, -5.8777)
  line L565 (32.8443, -5.8777) -> (31.878, -5.8777)
  line L566 (31.878, -5.8777) -> (31.878, -4.8028)
  line L567 (46.7019, -6.6012) -> (47.9163, -6.6012)
  line L568 (47.9163, -6.6012) -> (51.7507, -12.7507)
  line L569 (51.7507, -12.7507) -> (51.7507, -6.6012)
  line L570 (51.7507, -6.6012) -> (52.7273, -6.6012)
  line L571 (52.7273, -6.6012) -> (52.7273, -14.1924)
  line L572 (52.7273, -14.1924) -> (51.575, -14.1924)
  line L573 (51.575, -14.1924) -> (47.6837, -8.0481)
  line L574 (47.6837, -8.0481) -> (47.6837, -14.1924)
  line L575 (47.6837, -14.1924) -> (46.7019, -14.1924)
  line L576 (46.7019, -14.1924) -> (46.7019, -6.6012)
  line L577 (64.0579, -6.6012) -> (69.3237, -6.6012)
  line L578 (69.3237, -6.6012) -> (69.3237, -7.5313)
  line L579 (69.3237, -7.5313) -> (65.0863, -7.5313)
  line L580 (65.0863, -7.5313) -> (65.0863, -9.8361)
  line L581 (65.0863, -9.8361) -> (68.8122, -9.8361)
  line L582 (68.8122, -9.8361) -> (68.8122, -10.7405)
  line L583 (68.8122, -10.7405) -> (65.0863, -10.7405)
  line L584 (65.0863, -10.7405) -> (65.0863, -14.1924)
  line L585 (65.0863, -14.1924) -> (64.0579, -14.1924)
  line L586 (64.0579, -14.1924) -> (64.0579, -6.6012)
  line L587 (80.983, -14.1924) -> (79.7427, -14.1924)
  line L588 (79.7427, -14.1924) -> (82.4609, -10.3012)
  line L589 (82.4609, -10.3012) -> (79.9133, -6.6012)
  line L590 (79.9133, -6.6012) -> (81.2, -6.6012)
  line L591 (81.2, -6.6012) -> (83.1379, -9.5054)
  line L592 (83.1379, -9.5054) -> (85.0603, -6.6012)
  line L593 (85.0603, -6.6012) -> (86.285, -6.6012)
  line L594 (86.285, -6.6012) -> (83.7373, -10.3012)
  line L595 (83.7373, -10.3012) -> (86.409, -14.1924)
  line L596 (86.409, -14.1924) -> (85.1326, -14.1924)
  line L597 (85.1326, -14.1924) -> (83.0862, -11.0712)
  line L598 (83.0862, -11.0712) -> (80.983, -14.1924)
  line L599 (-86.6223, -31.8399) -> (-81.9662, -26.0057)
  line L600 (-81.9662, -26.0057) -> (-86.2812, -26.0057)
  line L601 (-86.2812, -26.0057) -> (-86.2812, -25.1013)
  line L602 (-86.2812, -25.1013) -> (-80.6433, -25.1013)
  line L603 (-80.6433, -25.1013) -> (-80.6433, -25.985)
  line L604 (-80.6433, -25.985) -> (-85.3252, -31.7883)
  line L605 (-85.3252, -31.7883) -> (-80.6433, -31.7883)
  line L606 (-80.6433, -31.7883) -> (-80.6433, -32.6926)
  line L607 (-80.6433, -32.6926) -> (-86.6223, -32.6926)
  line L608 (-86.6223, -32.6926) -> (-86.6223, -31.8399)
  line L609 (-69.5887, -25.1013) -> (-64.0542, -25.1013)
  line L610 (-64.0542, -25.1013) -> (-64.0542, -26.0315)
  line L611 (-64.0542, -26.0315) -> (-68.5862, -26.0315)
  line L612 (-68.5862, -26.0315) -> (-68.5862, -28.3363)
  line L613 (-68.5862, -28.3363) -> (-64.3952, -28.3363)
  line L614 (-64.3952, -28.3363) -> (-64.3952, -29.2148)
  line L615 (-64.3952, -29.2148) -> (-68.5862, -29.2148)
  line L616 (-68.5862, -29.2148) -> (-68.5862, -31.7883)
  line L617 (-68.5862, -31.7883) -> (-63.9766, -31.7883)
  line L618 (-63.9766, -31.7883) -> (-63.9766, -32.6926)
  line L619 (-63.9766, -32.6926) -> (-69.5887, -32.6926)
  line L620 (-69.5887, -32.6926) -> (-69.5887, -25.1013)
  line L621 (-53.2848, -25.1013) -> (-52.2461, -25.1013)
  line L622 (-52.2461, -25.1013) -> (-52.2461, -28.2381)
  line L623 (-52.2461, -28.2381) -> (-48.298, -28.2381)
  line L624 (-48.298, -28.2381) -> (-48.298, -25.1013)
  line L625 (-48.298, -25.1013) -> (-47.2593, -25.1013)
  line L626 (-47.2593, -25.1013) -> (-47.2593, -32.6926)
  line L627 (-47.2593, -32.6926) -> (-48.298, -32.6926)
  line L628 (-48.298, -32.6926) -> (-48.298, -29.1424)
  line L629 (-48.298, -29.1424) -> (-52.2461, -29.1424)
  line L630 (-52.2461, -29.1424) -> (-52.2461, -32.6926)
  line L631 (-52.2461, -32.6926) -> (-53.2848, -32.6926)
  line L632 (-53.2848, -32.6926) -> (-53.2848, -25.1013)
  line L633 (-36.6419, -25.1013) -> (-35.4275, -25.1013)
  line L634 (-35.4275, -25.1013) -> (-31.5931, -31.2508)
  line L635 (-31.5931, -31.2508) -> (-31.5931, -25.1013)
  line L636 (-31.5931, -25.1013) -> (-30.6164, -25.1013)
  line L637 (-30.6164, -25.1013) -> (-30.6164, -32.6926)
  line L638 (-30.6164, -32.6926) -> (-31.7688, -32.6926)
  line L639 (-31.7688, -32.6926) -> (-35.66, -26.5483)
  line L640 (-35.66, -26.5483) -> (-35.66, -32.6926)
  line L641 (-35.66, -32.6926) -> (-36.6419, -32.6926)
  line L642 (-36.6419, -32.6926) -> (-36.6419, -25.1013)
  line L643 (-19.5825, -25.1013) -> (-14.0479, -25.1013)
  line L644 (-14.0479, -25.1013) -> (-14.0479, -26.0315)
  line L645 (-14.0479, -26.0315) -> (-18.5799, -26.0315)
  line L646 (-18.5799, -26.0315) -> (-18.5799, -28.3363)
  line L647 (-18.5799, -28.3363) -> (-14.389, -28.3363)
  line L648 (-14.389, -28.3363) -> (-14.389, -29.2148)
  line L649 (-14.389, -29.2148) -> (-18.5799, -29.2148)
  line L650 (-18.5799, -29.2148) -> (-18.5799, -31.7883)
  line L651 (-18.5799, -31.7883) -> (-13.9704, -31.7883)
  line L652 (-13.9704, -31.7883) -> (-13.9704, -32.6926)
  line L653 (-13.9704, -32.6926) -> (-19.5825, -32.6926)
  line L654 (-19.5825, -32.6926) -> (-19.5825, -25.1013)
  line L655 (-2.1882, -25.1013) -> (-2.1882, -29.7936)
  spline S302 degree 3 poles (-2.1882, -29.7936) (-2.1882, -30.3444) (-2.0848, -30.8033) (-1.8781, -31.1681) knots 0 0 0 0 1 1 1 1
  spline S303 degree 3 poles (-1.8781, -31.1681) (-1.5712, -31.719) (-1.0544, -31.995) (-0.3278, -31.995) knots 0 0 0 0 1 1 1 1
  spline S304 degree 3 poles (-0.3278, -31.995) (0.5434, -31.995) (1.1367, -31.6973) (1.4499, -31.101) knots 0 0 0 0 1 1 1 1
  spline S305 degree 3 poles (1.4499, -31.101) (1.6183, -30.7775) (1.7031, -30.3413) (1.7031, -29.7936) knots 0 0 0 0 1 1 1 1
  line L656 (1.7031, -29.7936) -> (1.7031, -25.1013)
  line L657 (1.7031, -25.1013) -> (2.7469, -25.1013)
  line L658 (2.7469, -25.1013) -> (2.7469, -29.3646)
  spline S306 degree 3 poles (2.7469, -29.3646) (2.7469, -30.2979) (2.6208, -31.0162) (2.3697, -31.5195) knots 0 0 0 0 1 1 1 1
  spline S307 degree 3 poles (2.3697, -31.5195) (1.9077, -32.4363) (1.0364, -32.8941) (-0.2451, -32.8941) knots 0 0 0 0 1 1 1 1
  spline S308 degree 3 poles (-0.2451, -32.8941) (-1.5267, -32.8941) (-2.3969, -32.4363) (-2.8548, -31.5195) knots 0 0 0 0 1 1 1 1
  spline S309 degree 3 poles (-2.8548, -31.5195) (-3.1059, -31.0162) (-3.232, -30.2979) (-3.232, -29.3646) knots 0 0 0 0 1 1 1 1
  line L659 (-3.232, -29.3646) -> (-3.232, -25.1013)
  line L660 (-3.232, -25.1013) -> (-2.1882, -25.1013)
  line L661 (13.3644, -25.1013) -> (14.5788, -25.1013)
  line L662 (14.5788, -25.1013) -> (18.4132, -31.2508)
  line L663 (18.4132, -31.2508) -> (18.4132, -25.1013)
  line L664 (18.4132, -25.1013) -> (19.3898, -25.1013)
  line L665 (19.3898, -25.1013) -> (19.3898, -32.6926)
  line L666 (19.3898, -32.6926) -> (18.2375, -32.6926)
  line L667 (18.2375, -32.6926) -> (14.3462, -26.5483)
  line L668 (14.3462, -26.5483) -> (14.3462, -32.6926)
  line L669 (14.3462, -32.6926) -> (13.3644, -32.6926)
  line L670 (13.3644, -32.6926) -> (13.3644, -25.1013)
  spline S310 degree 3 poles (32.9477, -31.8141) (33.296, -31.8141) (33.5812, -31.7779) (33.8055, -31.7056) knots 0 0 0 0 1 1 1 1
  spline S311 degree 3 poles (33.8055, -31.7056) (34.2055, -31.5712) (34.5321, -31.3128) (34.7874, -30.9304) knots 0 0 0 0 1 1 1 1
  spline S312 degree 3 poles (34.7874, -30.9304) (34.991, -30.6235) (35.1367, -30.2307) (35.2266, -29.7522) knots 0 0 0 0 1 1 1 1
  spline S313 degree 3 poles (35.2266, -29.7522) (35.2783, -29.4659) (35.3041, -29.2013) (35.3041, -28.9564) knots 0 0 0 0 1 1 1 1
  spline S314 degree 3 poles (35.3041, -28.9564) (35.3041, -28.0159) (35.117, -27.2852) (34.7439, -26.7653) knots 0 0 0 0 1 1 1 1
  spline S315 degree 3 poles (34.7439, -26.7653) (34.3698, -26.2455) (33.7673, -25.985) (32.9373, -25.985) knots 0 0 0 0 1 1 1 1
  line L671 (32.9373, -25.985) -> (31.1132, -25.985)
  line L672 (31.1132, -25.985) -> (31.1132, -31.8141)
  line L673 (31.1132, -31.8141) -> (32.9477, -31.8141)
  line L674 (30.0796, -25.1013) -> (33.1544, -25.1013)
  spline S316 degree 3 poles (33.1544, -25.1013) (34.1982, -25.1013) (35.0075, -25.4713) (35.5832, -26.2124) knots 0 0 0 0 1 1 1 1
  spline S317 degree 3 poles (35.5832, -26.2124) (36.0968, -26.8811) (36.3531, -27.7368) (36.3531, -28.7807) knots 0 0 0 0 1 1 1 1
  spline S318 degree 3 poles (36.3531, -28.7807) (36.3531, -29.5868) (36.2012, -30.3155) (35.8984, -30.9666) knots 0 0 0 0 1 1 1 1
  spline S319 degree 3 poles (35.8984, -30.9666) (35.3641, -32.1169) (34.4463, -32.6926) (33.144, -32.6926) knots 0 0 0 0 1 1 1 1
  line L675 (33.144, -32.6926) -> (30.0796, -32.6926)
  line L676 (30.0796, -32.6926) -> (30.0796, -25.1013)
  spline S320 degree 3 poles (50.2314, -28.5792) (50.714, -28.5792) (51.0954, -28.483) (51.3755, -28.2898) knots 0 0 0 0 1 1 1 1
  spline S321 degree 3 poles (51.3755, -28.2898) (51.6566, -28.0965) (51.7972, -27.7492) (51.7972, -27.2459) knots 0 0 0 0 1 1 1 1
  spline S322 degree 3 poles (51.7972, -27.2459) (51.7972, -26.7054) (51.6008, -26.3364) (51.2081, -26.14) knots 0 0 0 0 1 1 1 1
  spline S323 degree 3 poles (51.2081, -26.14) (50.9983, -26.0367) (50.7171, -25.985) (50.3657, -25.985) knots 0 0 0 0 1 1 1 1
  line L677 (50.3657, -25.985) -> (47.8543, -25.985)
  line L678 (47.8543, -25.985) -> (47.8543, -28.5792)
  line L679 (47.8543, -28.5792) -> (50.2314, -28.5792)
  line L680 (46.8259, -25.1013) -> (50.3399, -25.1013)
  spline S324 degree 3 poles (50.3399, -25.1013) (50.9187, -25.1013) (51.3962, -25.1861) (51.7713, -25.3545) knots 0 0 0 0 1 1 1 1
  spline S325 degree 3 poles (51.7713, -25.3545) (52.4845, -25.678) (52.841, -26.2765) (52.841, -27.1477) knots 0 0 0 0 1 1 1 1
  spline S326 degree 3 poles (52.841, -27.1477) (52.841, -27.6025) (52.747, -27.9745) (52.5599, -28.2639) knots 0 0 0 0 1 1 1 1
  spline S327 degree 3 poles (52.5599, -28.2639) (52.3718, -28.5533) (52.1093, -28.7859) (51.7713, -28.9616) knots 0 0 0 0 1 1 1 1
  spline S328 degree 3 poles (51.7713, -28.9616) (52.068, -29.0825) (52.2912, -29.2406) (52.44, -29.437) knots 0 0 0 0 1 1 1 1
  spline S329 degree 3 poles (52.44, -29.437) (52.5899, -29.6334) (52.6736, -29.9517) (52.6912, -30.393) knots 0 0 0 0 1 1 1 1
  line L681 (52.6912, -30.393) -> (52.7273, -31.411)
  spline S330 degree 3 poles (52.7273, -31.411) (52.7377, -31.7004) (52.7615, -31.9154) (52.7997, -32.057) knots 0 0 0 0 1 1 1 1
  spline S331 degree 3 poles (52.7997, -32.057) (52.8617, -32.2978) (52.9723, -32.4528) (53.1304, -32.5221) knots 0 0 0 0 1 1 1 1
  line L682 (53.1304, -32.5221) -> (53.1304, -32.6926)
  line L683 (53.1304, -32.6926) -> (51.8695, -32.6926)
  spline S332 degree 3 poles (51.8695, -32.6926) (51.8354, -32.6275) (51.8075, -32.5427) (51.7868, -32.4394) knots 0 0 0 0 1 1 1 1
  spline S333 degree 3 poles (51.7868, -32.4394) (51.7662, -32.336) (51.7486, -32.1366) (51.7352, -31.8399) knots 0 0 0 0 1 1 1 1
  line L684 (51.7352, -31.8399) -> (51.6731, -30.5739)
  spline S334 degree 3 poles (51.6731, -30.5739) (51.6494, -30.0778) (51.4644, -29.745) (51.1202, -29.5765) knots 0 0 0 0 1 1 1 1
  spline S335 degree 3 poles (51.1202, -29.5765) (50.9238, -29.4835) (50.6158, -29.437) (50.1952, -29.437) knots 0 0 0 0 1 1 1 1
  line L685 (50.1952, -29.437) -> (47.8543, -29.437)
  line L686 (47.8543, -29.437) -> (47.8543, -32.6926)
  line L687 (47.8543, -32.6926) -> (46.8259, -32.6926)
  line L688 (46.8259, -32.6926) -> (46.8259, -25.1013)
  line L689 (63.7613, -25.1013) -> (69.2958, -25.1013)
  line L690 (69.2958, -25.1013) -> (69.2958, -26.0315)
  line L691 (69.2958, -26.0315) -> (64.7638, -26.0315)
  line L692 (64.7638, -26.0315) -> (64.7638, -28.3363)
  line L693 (64.7638, -28.3363) -> (68.9548, -28.3363)
  line L694 (68.9548, -28.3363) -> (68.9548, -29.2148)
  line L695 (68.9548, -29.2148) -> (64.7638, -29.2148)
  line L696 (64.7638, -29.2148) -> (64.7638, -31.7883)
  line L697 (64.7638, -31.7883) -> (69.3734, -31.7883)
  line L698 (69.3734, -31.7883) -> (69.3734, -32.6926)
  line L699 (69.3734, -32.6926) -> (63.7613, -32.6926)
  line L700 (63.7613, -32.6926) -> (63.7613, -25.1013)
  line L701 (82.6242, -25.1013) -> (83.6629, -25.1013)
  line L702 (83.6629, -25.1013) -> (83.6629, -32.6926)
  line L703 (83.6629, -32.6926) -> (82.6242, -32.6926)
  line L704 (82.6242, -32.6926) -> (82.6242, -25.1013)
  line L705 (-86.6223, -50.3401) -> (-81.9662, -44.5058)
  line L706 (-81.9662, -44.5058) -> (-86.2812, -44.5058)
  line L707 (-86.2812, -44.5058) -> (-86.2812, -43.6015)
  line L708 (-86.2812, -43.6015) -> (-80.6433, -43.6015)
  line L709 (-80.6433, -43.6015) -> (-80.6433, -44.4852)
  line L710 (-80.6433, -44.4852) -> (-85.3252, -50.2884)
  line L711 (-85.3252, -50.2884) -> (-80.6433, -50.2884)
  line L712 (-80.6433, -50.2884) -> (-80.6433, -51.1928)
  line L713 (-80.6433, -51.1928) -> (-86.6223, -51.1928)
  line L714 (-86.6223, -51.1928) -> (-86.6223, -50.3401)
  line L715 (-70.6501, -43.6015) -> (-69.2187, -49.7768)
  line L716 (-69.2187, -49.7768) -> (-67.503, -43.6015)
  line L717 (-67.503, -43.6015) -> (-66.3868, -43.6015)
  line L718 (-66.3868, -43.6015) -> (-64.6712, -49.7768)
  line L719 (-64.6712, -49.7768) -> (-63.2397, -43.6015)
  line L720 (-63.2397, -43.6015) -> (-62.1132, -43.6015)
  line L721 (-62.1132, -43.6015) -> (-64.1079, -51.1928)
  line L722 (-64.1079, -51.1928) -> (-65.1879, -51.1928)
  line L723 (-65.1879, -51.1928) -> (-66.9398, -44.8986)
  line L724 (-66.9398, -44.8986) -> (-68.7019, -51.1928)
  line L725 (-68.7019, -51.1928) -> (-69.782, -51.1928)
  line L726 (-69.782, -51.1928) -> (-71.7663, -43.6015)
  line L727 (-71.7663, -43.6015) -> (-70.6501, -43.6015)
  line L728 (-52.92, -43.6015) -> (-47.3854, -43.6015)
  line L729 (-47.3854, -43.6015) -> (-47.3854, -44.5317)
  line L730 (-47.3854, -44.5317) -> (-51.9174, -44.5317)
  line L731 (-51.9174, -44.5317) -> (-51.9174, -46.8364)
  line L732 (-51.9174, -46.8364) -> (-47.7265, -46.8364)
  line L733 (-47.7265, -46.8364) -> (-47.7265, -47.7149)
  line L734 (-47.7265, -47.7149) -> (-51.9174, -47.7149)
  line L735 (-51.9174, -47.7149) -> (-51.9174, -50.2884)
  line L736 (-51.9174, -50.2884) -> (-47.3079, -50.2884)
  line L737 (-47.3079, -50.2884) -> (-47.3079, -51.1928)
  line L738 (-47.3079, -51.1928) -> (-52.92, -51.1928)
  line L739 (-52.92, -51.1928) -> (-52.92, -43.6015)
  line L740 (-34.057, -43.6015) -> (-33.0183, -43.6015)
  line L741 (-33.0183, -43.6015) -> (-33.0183, -51.1928)
  line L742 (-33.0183, -51.1928) -> (-34.057, -51.1928)
  line L743 (-34.057, -51.1928) -> (-34.057, -43.6015)
  line L744 (-19.9731, -43.6015) -> (-18.7587, -43.6015)
  line L745 (-18.7587, -43.6015) -> (-14.9243, -49.751)
  line L746 (-14.9243, -49.751) -> (-14.9243, -43.6015)
  line L747 (-14.9243, -43.6015) -> (-13.9477, -43.6015)
  line L748 (-13.9477, -43.6015) -> (-13.9477, -51.1928)
  line L749 (-13.9477, -51.1928) -> (-15.1, -51.1928)
  line L750 (-15.1, -51.1928) -> (-18.9913, -45.0484)
  line L751 (-18.9913, -45.0484) -> (-18.9913, -51.1928)
  line L752 (-18.9913, -51.1928) -> (-19.9731, -51.1928)
  line L753 (-19.9731, -51.1928) -> (-19.9731, -43.6015)
  spline S336 degree 3 poles (-2.3401, -48.7433) (-2.3163, -49.1743) (-2.214, -49.5236) (-2.0352, -49.7923) knots 0 0 0 0 1 1 1 1
  spline S337 degree 3 poles (-2.0352, -49.7923) (-1.6941, -50.2957) (-1.0926, -50.5468) (-0.2317, -50.5468) knots 0 0 0 0 1 1 1 1
  spline S338 degree 3 poles (-0.2317, -50.5468) (0.1538, -50.5468) (0.5052, -50.492) (0.8225, -50.3814) knots 0 0 0 0 1 1 1 1
  spline S339 degree 3 poles (0.8225, -50.3814) (1.4354, -50.1675) (1.7423, -49.7851) (1.7423, -49.2342) knots 0 0 0 0 1 1 1 1
  spline S340 degree 3 poles (1.7423, -49.2342) (1.7423, -48.8208) (1.6132, -48.5263) (1.3548, -48.3506) knots 0 0 0 0 1 1 1 1
  spline S341 degree 3 poles (1.3548, -48.3506) (1.0933, -48.178) (0.683, -48.0281) (0.1249, -47.901) knots 0 0 0 0 1 1 1 1
  line L754 (0.1249, -47.901) -> (-0.9035, -47.6684)
  spline S342 degree 3 poles (-0.9035, -47.6684) (-1.5753, -47.5165) (-2.0507, -47.3501) (-2.3298, -47.1672) knots 0 0 0 0 1 1 1 1
  spline S343 degree 3 poles (-2.3298, -47.1672) (-2.8124, -46.8499) (-3.0532, -46.3765) (-3.0532, -45.7461) knots 0 0 0 0 1 1 1 1
  spline S344 degree 3 poles (-3.0532, -45.7461) (-3.0532, -45.0639) (-2.8176, -44.5038) (-2.3453, -44.0666) knots 0 0 0 0 1 1 1 1
  spline S345 degree 3 poles (-2.3453, -44.0666) (-1.8729, -43.6294) (-1.2053, -43.4103) (-0.3402, -43.4103) knots 0 0 0 0 1 1 1 1
  spline S346 degree 3 poles (-0.3402, -43.4103) (0.4556, -43.4103) (1.1315, -43.6025) (1.6886, -43.987) knots 0 0 0 0 1 1 1 1
  spline S347 degree 3 poles (1.6886, -43.987) (2.2446, -44.3704) (2.5227, -44.9844) (2.5227, -45.8288) knots 0 0 0 0 1 1 1 1
  line L755 (2.5227, -45.8288) -> (1.5563, -45.8288)
  spline S348 degree 3 poles (1.5563, -45.8288) (1.5046, -45.4226) (1.394, -45.1104) (1.2256, -44.8934) knots 0 0 0 0 1 1 1 1
  spline S349 degree 3 poles (1.2256, -44.8934) (0.9124, -44.4976) (0.3802, -44.2991) (-0.3712, -44.2991) knots 0 0 0 0 1 1 1 1
  spline S350 degree 3 poles (-0.3712, -44.2991) (-0.9779, -44.2991) (-1.413, -44.4263) (-1.6786, -44.6815) knots 0 0 0 0 1 1 1 1
  spline S351 degree 3 poles (-1.6786, -44.6815) (-1.9443, -44.9368) (-2.0765, -45.2324) (-2.0765, -45.5704) knots 0 0 0 0 1 1 1 1
  spline S352 degree 3 poles (-2.0765, -45.5704) (-2.0765, -45.9424) (-1.9215, -46.2143) (-1.6115, -46.3869) knots 0 0 0 0 1 1 1 1
  spline S353 degree 3 poles (-1.6115, -46.3869) (-1.4079, -46.4974) (-0.9479, -46.6349) (-0.2317, -46.8003) knots 0 0 0 0 1 1 1 1
  line L756 (-0.2317, -46.8003) -> (0.8328, -47.0431)
  spline S354 degree 3 poles (0.8328, -47.0431) (1.3465, -47.1599) (1.7423, -47.3201) (2.0214, -47.5237) knots 0 0 0 0 1 1 1 1
  spline S355 degree 3 poles (2.0214, -47.5237) (2.5041, -47.8782) (2.7449, -48.394) (2.7449, -49.0689) knots 0 0 0 0 1 1 1 1
  spline S356 degree 3 poles (2.7449, -49.0689) (2.7449, -49.9091) (2.4389, -50.5106) (1.8271, -50.8724) knots 0 0 0 0 1 1 1 1
  spline S357 degree 3 poles (1.8271, -50.8724) (1.2163, -51.2341) (0.5052, -51.415) (-0.304, -51.415) knots 0 0 0 0 1 1 1 1
  spline S358 degree 3 poles (-0.304, -51.415) (-1.2477, -51.415) (-1.9866, -51.1742) (-2.521, -50.6915) knots 0 0 0 0 1 1 1 1
  spline S359 degree 3 poles (-2.521, -50.6915) (-3.0553, -50.213) (-3.3168, -49.5629) (-3.3064, -48.7433) knots 0 0 0 0 1 1 1 1
  line L757 (-3.3064, -48.7433) -> (-2.3401, -48.7433)
  line L758 (15.9492, -43.6015) -> (16.9879, -43.6015)
  line L759 (16.9879, -43.6015) -> (16.9879, -51.1928)
  line L760 (16.9879, -51.1928) -> (15.9492, -51.1928)
  line L761 (15.9492, -51.1928) -> (15.9492, -43.6015)
  line L762 (30.4238, -43.6015) -> (35.9583, -43.6015)
  line L763 (35.9583, -43.6015) -> (35.9583, -44.5317)
  line L764 (35.9583, -44.5317) -> (31.4263, -44.5317)
  line L765 (31.4263, -44.5317) -> (31.4263, -46.8364)
  line L766 (31.4263, -46.8364) -> (35.6173, -46.8364)
  line L767 (35.6173, -46.8364) -> (35.6173, -47.7149)
  line L768 (35.6173, -47.7149) -> (31.4263, -47.7149)
  line L769 (31.4263, -47.7149) -> (31.4263, -50.2884)
  line L770 (31.4263, -50.2884) -> (36.0359, -50.2884)
  line L771 (36.0359, -50.2884) -> (36.0359, -51.1928)
  line L772 (36.0359, -51.1928) -> (30.4238, -51.1928)
  line L773 (30.4238, -51.1928) -> (30.4238, -43.6015)
  spline S360 degree 3 poles (49.8469, -46.8106) (50.281, -46.8106) (50.6189, -46.7507) (50.8598, -46.6297) knots 0 0 0 0 1 1 1 1
  spline S361 degree 3 poles (50.8598, -46.6297) (51.2391, -46.4406) (51.4282, -46.0995) (51.4282, -45.6065) knots 0 0 0 0 1 1 1 1
  spline S362 degree 3 poles (51.4282, -45.6065) (51.4282, -45.1104) (51.2267, -44.7766) (50.8236, -44.604) knots 0 0 0 0 1 1 1 1
  spline S363 degree 3 poles (50.8236, -44.604) (50.5962, -44.5079) (50.2582, -44.4593) (49.8107, -44.4593) knots 0 0 0 0 1 1 1 1
  line L774 (49.8107, -44.4593) -> (47.9762, -44.4593)
  line L775 (47.9762, -44.4593) -> (47.9762, -46.8106)
  line L776 (47.9762, -46.8106) -> (49.8469, -46.8106)
  spline S364 degree 3 poles (50.1931, -50.3143) (50.8236, -50.3143) (51.2732, -50.1313) (51.5419, -49.7665) knots 0 0 0 0 1 1 1 1
  spline S365 degree 3 poles (51.5419, -49.7665) (51.7104, -49.536) (51.7951, -49.257) (51.7951, -48.9293) knots 0 0 0 0 1 1 1 1
  spline S366 degree 3 poles (51.7951, -48.9293) (51.7951, -48.3785) (51.5491, -48.0023) (51.0561, -47.8028) knots 0 0 0 0 1 1 1 1
  spline S367 degree 3 poles (51.0561, -47.8028) (50.7946, -47.6963) (50.4484, -47.6426) (50.0174, -47.6426) knots 0 0 0 0 1 1 1 1
  line L777 (50.0174, -47.6426) -> (47.9762, -47.6426)
  line L778 (47.9762, -47.6426) -> (47.9762, -50.3143)
  line L779 (47.9762, -50.3143) -> (50.1931, -50.3143)
  line L780 (46.9685, -43.6015) -> (50.2293, -43.6015)